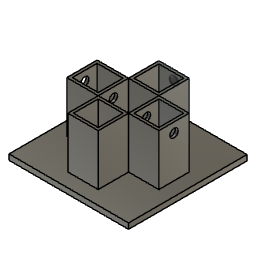
button_set (Autodesk Fusion 360 design; units mm, degrees)
Autodesk Fusion 360 part; units mm, degrees
sketch "Sketch1" plane through (0, 0, 0) normal (0, 0, 1) x (1, 0, 0)
  line L0 (0, 0) -> (11.4, 0)
  line L1 (11.4, 0) -> (11.4, 11)
  line L2 (11.4, 11) -> (0, 11)
  line L3 (0, 11) -> (0, 0)
  line L4 (11.4, 0) -> (22.4, 0)
  line L5 (22.4, 0) -> (22.4, -11)
  line L6 (22.4, -11) -> (11.4, -11)
  line L7 (11.4, -11) -> (11.4, 0)
  line L8 (22.4, 0) -> (33.4, 0)
  line L9 (33.4, 0) -> (33.4, 11)
  line L10 (33.4, 11) -> (22.4, 11)
  line L11 (22.4, 11) -> (22.4, 0)
  line L12 (11.4, 11) -> (22.4, 11)
  line L13 (22.4, 11) -> (22.4, 22)
  line L14 (22.4, 22) -> (11.4, 22)
  line L15 (11.4, 22) -> (11.4, 11)
  line L16 (1, 10) -> (10.4, 10)
  line L17 (10.4, 10) -> (10.4, 1)
  line L18 (10.4, 1) -> (1, 1)
  line L19 (1, 1) -> (1, 10)
  line L20 (33.4, -11.0012) -> (0, -11.0012)
  line L21 (0, -11.0012) -> (0, 22)
  line L22 (0, 22) -> (33.4, 22)
  line L23 (33.4, 22) -> (33.4, -11.0012)
  line L24 (12.4, -1) -> (21.4, -1)
  line L25 (21.4, -1) -> (21.4, -10)
  line L26 (21.4, -10) -> (12.4, -10)
  line L27 (12.4, -10) -> (12.4, -1)
  line L28 (23.4, 10) -> (32.4, 10)
  line L29 (32.4, 10) -> (32.4, 1)
  line L30 (32.4, 1) -> (23.4, 1)
  line L31 (23.4, 1) -> (23.4, 10)
  line L32 (12.4, 21) -> (21.4, 21)
  line L33 (21.4, 21) -> (21.4, 12)
  line L34 (21.4, 12) -> (12.4, 12)
  line L35 (12.4, 12) -> (12.4, 21)
  circle A0 centre (16.9, -5.5) radius 3.5
  circle A1 centre (27.9, 5.5) radius 3.5
  circle A2 centre (16.9, 16.5) radius 3.5
  circle A3 centre (5.5, 5.5) radius 3.5
  line L36 (-5, 27) -> (38.4, 27)
  line L37 (38.4, 27) -> (38.4, -16.0012)
  line L38 (38.4, -16.0012) -> (-5, -16.0012)
  line L39 (-5, -16.0012) -> (-5, 27)
  dimension "d1" = 11.4
  dimension "d2" = 11
  dimension "d3" = 11
  dimension "d4" = 11
  dimension "d5" = 11
  dimension "d6" = 11
  dimension "d7" = 11
  dimension "d8" = 11
  dimension "d9" = 1
  dimension "d10" = 1
  dimension "d11" = 1
  dimension "d12" = 1
  dimension "d13" = 1
  dimension "d14" = 1
  dimension "d15" = 1
  dimension "d16" = 1
  dimension "d17" = 1
  dimension "d18" = 1
  dimension "d19" = 1
  dimension "d20" = 1
  dimension "d21" = 1
  dimension "d22" = 1
  dimension "d23" = 1
  dimension "d24" = 1
  dimension "d25" = 1
  dimension "d26" = 7
  dimension "d27" = 4.5
  dimension "d28" = 4.5
  dimension "d29" = 7
  dimension "d30" = 4.5
  dimension "d31" = 4.5
  dimension "d32" = 7
  dimension "d33" = 7
  dimension "d34" = 4.5
  dimension "d35" = 4.5
  dimension "d36" = 4.5
  dimension "d37" = 4.5
  dimension "d38" = 5
  dimension "d39" = 5
  dimension "d40" = 5
  dimension "d41" = 5
  constraint horizontal L0
  constraint vertical L1
  constraint horizontal L2
  constraint vertical L3
  constraint coincident L0.start L3.end
  constraint horizontal L4
  constraint vertical L5
  constraint horizontal L6
  constraint vertical L7
  constraint horizontal L8
  constraint vertical L9
  constraint horizontal L10
  constraint vertical L11
  constraint horizontal L12
  constraint vertical L13
  constraint horizontal L14
  constraint vertical L15
  constraint horizontal L16
  constraint vertical L17
  constraint horizontal L18
  constraint vertical L19
  constraint horizontal L20
  constraint vertical L21
  constraint horizontal L22
  constraint vertical L23
  constraint horizontal L24
  constraint vertical L25
  constraint horizontal L26
  constraint vertical L27
  constraint horizontal L28
  constraint vertical L29
  constraint horizontal L30
  constraint vertical L31
  constraint horizontal L32
  constraint vertical L33
  constraint horizontal L34
  constraint vertical L35
  constraint horizontal L36
  constraint vertical L37
  constraint horizontal L38
  constraint vertical L39
  measures "d1" distance of L0.start L0.end
  measures "d2" distance of L0.start L2.end
  measures "d3" distance of L0.end L4.end
  measures "d4" distance of L0.end L6.end
  measures "d5" distance of L4.end L8.end
  measures "d6" distance of L4.end L10.end
  measures "d7" distance of L1.end L10.end
  measures "d8" distance of L1.end L14.end
  measures "d9" distance of L2 L16
  measures "d10" distance of L3 L19
  measures "d11" distance of L1 L17
  measures "d12" distance of L0 L18
  measures "d13" distance of L14 L32
  measures "d14" distance of L15 L35
  measures "d15" distance of L13 L33
  measures "d16" distance of L12 L34
  measures "d17" distance of L23 L29
  measures "d18" distance of L10 L28
  measures "d19" distance of L8 L30
  measures "d20" distance of L11 L31
  measures "d21" distance of L9 L29
  measures "d22" distance of L5 L25
  measures "d23" distance of L4 L24
  measures "d24" distance of L7 L27
  measures "d25" distance of L6 L26
  measures "d26" diameter of A0
  measures "d27" distance of L24 A0.centre
  measures "d28" distance of L27 A0.centre
  measures "d29" diameter of A1
  measures "d30" distance of L28 A1.centre
  measures "d31" distance of L31 A1.centre
  measures "d32" diameter of A2
  measures "d33" diameter of A3
  measures "d34" distance of L35 A2.centre
  measures "d35" distance of L32 A2.centre
  measures "d36" distance of L16 A3.centre
  measures "d37" distance of L19 A3.centre
  measures "d38" distance of L22 L36
  measures "d39" distance of L21 L39
  measures "d40" distance of L20 L38
  measures "d41" distance of L23 L37
extrude "Extrude1" add sketch "Sketch1" along normal blind 2 contours L0 L7 L20 L21 | L1 L4 L11 L12 | L2 L15 L21 L22 | L5 L8 L20 L23 | L10 L13 L22 L23 | L36 L37 L38 L39 makes body 1
extrude "Extrude2" add sketch "Sketch1" along normal blind 15.5 separate body contours L0 L1 L2 L3 L21 | L4 L5 L6 L7 L20 | L12 L13 L14 L15 L22 | L8 L9 L10 L11 L23 makes body 2
extrude "Extrude3" add sketch "Sketch1" along normal blind 6.5 separate body contours L16 L17 L18 L19 | L24 L25 L26 L27 | L28 L29 L30 L31 | L32 L33 L34 L35 makes body 3 at (8.9826, 5.1515, 4.3333) makes body 4 at (20.3826, 16.1515, 4.3333) makes body 5 at (20.3826, -5.8485, 4.3333) makes body 6 at (31.3826, 5.1515, 4.3333)
extrude "Extrude4" add 4 faces at (4.1333, 0.3333, 15.5) (22.0667, 15, 15.5) (26.4, 0.3333, 15.5) (15.4, -0.3333, 15.5) along direction (0, 0, 1) blind 5 on bodies 2 bodies 2
sketch "Sketch2" plane through (33.4, 0, 0) normal (1, 0, 0) x (0, 1, 0)
  line L0 (0, 0) -> (11, 0)
  line L1 (11, 0) -> (11, 20.5)
  line L2 (11, 20.5) -> (0, 20.5)
  line L3 (0, 20.5) -> (0, 0)
  circle A0 centre (5.5, 17) radius 1.5
  dimension "d50" = 3
  dimension "d51" = 3.5
  dimension "d52" = 5.5
  measures "d50" diameter of A0
  measures "d51" distance of L2 A0.centre
  measures "d52" distance of L3 A0.centre
extrude "Extrude5" cut sketch "Sketch2" against normal blind 53 contours A0 bodies 2
sketch "Sketch3" plane through (0, 22, 0) normal (0, 1, 0) x (-1, 0, 0)
  line L0 (-22.4, 0) -> (-11.4, 0)
  line L1 (-11.4, 0) -> (-11.4, 20.5)
  line L2 (-11.4, 20.5) -> (-22.4, 20.5)
  line L3 (-22.4, 20.5) -> (-22.4, 0)
  circle A0 centre (-16.9, 17) radius 1.5
  dimension "d55" = 3
  dimension "d56" = 3.5
  dimension "d57" = 5.5
  measures "d55" diameter of A0
  measures "d56" distance of L2 A0.centre
  measures "d57" distance of L3 A0.centre
copy_body "Body->Comp1" bodies 1 removing the originals makes body 7 in component "Component"
copy_body "CutPasteBodies1" bodies 2 removing the originals makes body 8 in component "Component"
copy_body "CutPasteBodies2" bodies 3 removing the originals makes body 9 in component "Component"
copy_body "CutPasteBodies3" bodies 4 removing the originals makes body 10 in component "Component"
copy_body "CutPasteBodies4" bodies 5 removing the originals makes body 11 in component "Component"
copy_body "CutPasteBodies5" bodies 6 removing the originals makes body 12 in component "Component"
component "Component" placed x (1, 0, 0) y (0, 1, 0) z (0, 0, 1) at (0, 0, 0)
